Autodesk Inventor part; units mm, degrees
(part 2 of 2)
  spline S266 degree 2 poles (0.3678, -0.7093) (0.2402, -0.5675) (0.1065, -0.294) (0.1065, -0.14) knots 0 0 0 1 2 2 2
  spline S267 degree 2 poles (0.1065, -0.14) (0.1065, 0.1355) (0.4712, 0.4475) (0.8176, 0.4475) knots 0 0 0 1 2 2 2
  line L239 (0.8176, 0.4475) -> (2.0352, 0.4475)
  line L240 (2.831, -11.0699) -> (2.831, -12.2328)
  line L241 (2.831, -12.2328) -> (3.536, -12.2328)
  line L242 (3.536, -12.2328) -> (3.536, -11.1185)
  line L243 (3.536, -11.1185) -> (3.8318, -11.1185)
  line L244 (3.8318, -11.1185) -> (3.8318, -12.2328)
  line L245 (3.8318, -12.2328) -> (5.0352, -12.2328)
  line L246 (5.0352, -12.2328) -> (5.0352, -12.565)
  line L247 (5.0352, -12.565) -> (2.5352, -12.565)
  line L248 (2.5352, -12.565) -> (2.5352, -11.0699)
  line L249 (2.5352, -11.0699) -> (2.831, -11.0699)
  line L250 (5.0352, -10.4743) -> (5.0352, -10.7903)
  line L251 (5.0352, -10.7903) -> (3.1592, -10.7903)
  line L252 (3.1592, -10.7903) -> (3.1592, -10.4743)
  line L253 (3.1592, -10.4743) -> (5.0352, -10.4743)
  line L254 (2.8472, -10.452) -> (2.8472, -10.8106)
  line L255 (2.8472, -10.8106) -> (2.519, -10.8106)
  line L256 (2.519, -10.8106) -> (2.519, -10.452)
  line L257 (2.519, -10.452) -> (2.8472, -10.452)
  line L258 (5.0352, -9.6882) -> (5.0352, -10.0043)
  line L259 (5.0352, -10.0043) -> (2.4238, -10.0043)
  line L260 (2.4238, -10.0043) -> (2.4238, -9.6882)
  line L261 (2.4238, -9.6882) -> (5.0352, -9.6882)
  line L262 (5.0352, -8.9022) -> (5.0352, -9.2182)
  line L263 (5.0352, -9.2182) -> (3.1592, -9.2182)
  line L264 (3.1592, -9.2182) -> (3.1592, -8.9022)
  line L265 (3.1592, -8.9022) -> (5.0352, -8.9022)
  line L266 (2.8472, -8.8799) -> (2.8472, -9.2385)
  line L267 (2.8472, -9.2385) -> (2.519, -9.2385)
  line L268 (2.519, -9.2385) -> (2.519, -8.8799)
  line L269 (2.519, -8.8799) -> (2.8472, -8.8799)
  spline S268 degree 2 poles (4.0465, -6.8661) (4.5165, -6.8661) (5.0716, -7.3138) (5.0716, -7.6562) knots 0 0 0 1 2 2 2
  spline S269 degree 2 poles (5.0716, -7.6562) (5.0716, -7.796) (5.0068, -8.0108) (4.94, -8.1222) knots 0 0 0 1 2 2 2
  line L270 (4.94, -8.1222) -> (5.726, -8.1222)
  line L271 (5.726, -8.1222) -> (5.726, -8.4382)
  line L272 (5.726, -8.4382) -> (3.1592, -8.4382)
  line L273 (3.1592, -8.4382) -> (3.1592, -8.1222)
  line L274 (3.1592, -8.1222) -> (3.3557, -8.1222)
  spline S270 degree 2 poles (3.3557, -8.1222) (3.2483, -8.0047) (3.1065, -7.717) (3.1065, -7.5488) knots 0 0 0 1 2 2 2
  spline S271 degree 2 poles (3.1065, -7.5488) (3.1065, -7.2267) (3.617, -6.8661) (4.0465, -6.8661) knots 0 0 0 1 2 2 2
  spline S272 degree 2 poles (4.083, -7.1923) (3.7609, -7.1923) (3.4063, -7.3969) (3.4063, -7.6258) knots 0 0 0 1 2 2 2
  spline S273 degree 2 poles (3.4063, -7.6258) (3.4063, -7.7595) (3.5259, -8.0108) (3.6191, -8.1222) knots 0 0 0 1 2 2 2
  line L275 (3.6191, -8.1222) -> (4.6847, -8.1222)
  spline S274 degree 2 poles (4.6847, -8.1222) (4.7434, -7.9986) (4.788, -7.8223) (4.788, -7.7089) knots 0 0 0 1 2 2 2
  spline S275 degree 2 poles (4.788, -7.7089) (4.788, -7.4638) (4.4274, -7.1923) (4.083, -7.1923) knots 0 0 0 1 2 2 2
  line L276 (5.0352, -4.984) -> (5.0352, -5.3993)
  line L277 (5.0352, -5.3993) -> (4.1296, -6.0962)
  line L278 (4.1296, -6.0962) -> (4.2511, -6.2219)
  line L279 (4.2511, -6.2219) -> (5.0352, -6.2219)
  line L280 (5.0352, -6.2219) -> (5.0352, -6.5379)
  line L281 (5.0352, -6.5379) -> (2.4238, -6.5379)
  line L282 (2.4238, -6.5379) -> (2.4238, -6.2219)
  line L283 (2.4238, -6.2219) -> (3.9513, -6.2219)
  line L284 (3.9513, -6.2219) -> (3.1592, -5.4804)
  line L285 (3.1592, -5.4804) -> (3.1592, -5.0873)
  line L286 (3.1592, -5.0873) -> (3.9432, -5.8572)
  line L287 (3.9432, -5.8572) -> (5.0352, -4.984)
  spline S276 degree 2 poles (4.0972, -3.2843) (4.5712, -3.2843) (5.0879, -3.7401) (5.0879, -4.121) knots 0 0 0 1 2 2 2
  spline S277 degree 2 poles (5.0879, -4.121) (5.0879, -4.512) (4.555, -4.9597) (4.0972, -4.9597) knots 0 0 0 1 2 2 2
  spline S278 degree 2 poles (4.0972, -4.9597) (3.6272, -4.9597) (3.1065, -4.4978) (3.1065, -4.121) knots 0 0 0 1 2 2 2
  spline S279 degree 2 poles (3.1065, -4.121) (3.1065, -3.7401) (3.6251, -3.2843) (4.0972, -3.2843) knots 0 0 0 1 2 2 2
  spline S280 degree 2 poles (4.0972, -3.6104) (3.7325, -3.6104) (3.378, -3.8758) (3.378, -4.121) knots 0 0 0 1 2 2 2
  spline S281 degree 2 poles (3.378, -4.121) (3.378, -4.3661) (3.7325, -4.6335) (4.0972, -4.6335) knots 0 0 0 1 2 2 2
  spline S282 degree 2 poles (4.0972, -4.6335) (4.4517, -4.6335) (4.8164, -4.3661) (4.8164, -4.121) knots 0 0 0 1 2 2 2
  spline S283 degree 2 poles (4.8164, -4.121) (4.8164, -3.8779) (4.4578, -3.6104) (4.0972, -3.6104) knots 0 0 0 1 2 2 2
  line L288 (3.1592, -0.687) -> (5.0352, -1.1631)
  line L289 (5.0352, -1.1631) -> (5.0352, -1.4548)
  line L290 (5.0352, -1.4548) -> (3.5887, -1.9127)
  line L291 (3.5887, -1.9127) -> (5.0352, -2.3685)
  line L292 (5.0352, -2.3685) -> (5.0352, -2.6582)
  line L293 (5.0352, -2.6582) -> (3.1592, -3.1384)
  line L294 (3.1592, -3.1384) -> (3.1592, -2.8102)
  line L295 (3.1592, -2.8102) -> (4.6118, -2.4779)
  line L296 (4.6118, -2.4779) -> (3.1592, -2.0343)
  line L297 (3.1592, -2.0343) -> (3.1592, -1.7729)
  line L298 (3.1592, -1.7729) -> (4.6118, -1.3171)
  line L299 (4.6118, -1.3171) -> (3.1592, -1.0051)
  line L300 (3.1592, -1.0051) -> (3.1592, -0.687)
  spline S284 degree 2 poles (5.0797, 0.097) (5.0797, -0.0914) (4.9785, -0.4176) (4.9217, -0.5249) knots 0 0 0 1 2 2 2
  line L301 (4.9217, -0.5249) -> (4.5672, -0.5249)
  line L302 (4.5672, -0.5249) -> (4.5672, -0.5087)
  spline S285 degree 2 poles (4.5672, -0.5087) (4.5996, -0.4682) (4.6766, -0.3588) (4.7191, -0.2676) knots 0 0 0 1 2 2 2
  spline S286 degree 2 poles (4.7191, -0.2676) (4.7576, -0.1886) (4.8144, 0.0059) (4.8144, 0.1092) knots 0 0 0 1 2 2 2
  spline S287 degree 2 poles (4.8144, 0.1092) (4.8144, 0.1841) (4.7799, 0.3563) (4.7515, 0.3969) knots 0 0 0 1 2 2 2
  spline S288 degree 2 poles (4.7515, 0.3969) (4.7131, 0.4556) (4.6259, 0.5083) (4.5368, 0.5083) knots 0 0 0 1 2 2 2
  spline S289 degree 2 poles (4.5368, 0.5083) (4.4254, 0.5083) (4.3099, 0.3867) (4.2714, 0.2307) knots 0 0 0 1 2 2 2
  spline S290 degree 2 poles (4.2714, 0.2307) (4.2572, 0.17) (4.2167, -0.0245) (4.1944, -0.1076) knots 0 0 0 1 2 2 2
  spline S291 degree 2 poles (4.1944, -0.1076) (4.1316, -0.3223) (3.8723, -0.5168) (3.6879, -0.5168) knots 0 0 0 1 2 2 2
  spline S292 degree 2 poles (3.6879, -0.5168) (3.4327, -0.5168) (3.1146, -0.1339) (3.1146, 0.1821) knots 0 0 0 1 2 2 2
  spline S293 degree 2 poles (3.1146, 0.1821) (3.1146, 0.3381) (3.1916, 0.6542) (3.2503, 0.7615) knots 0 0 0 1 2 2 2
  line L303 (3.2503, 0.7615) -> (3.5887, 0.7615)
  line L304 (3.5887, 0.7615) -> (3.5887, 0.7453)
  spline S294 degree 2 poles (3.5887, 0.7453) (3.4914, 0.6238) (3.38, 0.328) (3.38, 0.176) knots 0 0 0 1 2 2 2
  spline S295 degree 2 poles (3.38, 0.176) (3.38, 0.02) (3.5117, -0.1947) (3.6434, -0.1947) knots 0 0 0 1 2 2 2
  spline S296 degree 2 poles (3.6434, -0.1947) (3.7629, -0.1947) (3.8784, -0.0671) (3.9148, 0.0747) knots 0 0 0 1 2 2 2
  spline S297 degree 2 poles (3.9148, 0.0747) (3.9331, 0.1436) (3.9695, 0.3179) (3.9918, 0.4131) knots 0 0 0 1 2 2 2
  spline S298 degree 2 poles (3.9918, 0.4131) (4.0445, 0.6197) (4.2856, 0.8304) (4.4943, 0.8304) knots 0 0 0 1 2 2 2
  spline S299 degree 2 poles (4.4943, 0.8304) (4.6158, 0.8304) (4.8306, 0.7352) (4.9096, 0.642) knots 0 0 0 1 2 2 2
  spline S300 degree 2 poles (4.9096, 0.642) (4.9926, 0.5427) (5.0797, 0.2895) (5.0797, 0.097) knots 0 0 0 1 2 2 2
  line L305 (5.0352, 2.6781) -> (5.0352, 2.2627)
  line L306 (5.0352, 2.2627) -> (4.1296, 1.5658)
  line L307 (4.1296, 1.5658) -> (4.2511, 1.4402)
  line L308 (4.2511, 1.4402) -> (5.0352, 1.4402)
  line L309 (5.0352, 1.4402) -> (5.0352, 1.1242)
  line L310 (5.0352, 1.1242) -> (2.4238, 1.1242)
  line L311 (2.4238, 1.1242) -> (2.4238, 1.4402)
  line L312 (2.4238, 1.4402) -> (3.9513, 1.4402)
  line L313 (3.9513, 1.4402) -> (3.1592, 2.1817)
  line L314 (3.1592, 2.1817) -> (3.1592, 2.5747)
  line L315 (3.1592, 2.5747) -> (3.9432, 1.8049)
  line L316 (3.9432, 1.8049) -> (5.0352, 2.6781)
  line L317 (5.0352, 3.1582) -> (5.0352, 2.8422)
  line L318 (5.0352, 2.8422) -> (3.1592, 2.8422)
  line L319 (3.1592, 2.8422) -> (3.1592, 3.1582)
  line L320 (3.1592, 3.1582) -> (5.0352, 3.1582)
  line L321 (2.8472, 3.1805) -> (2.8472, 2.8219)
  line L322 (2.8472, 2.8219) -> (2.519, 2.8219)
  line L323 (2.519, 2.8219) -> (2.519, 3.1805)
  line L324 (2.519, 3.1805) -> (2.8472, 3.1805)
  line L325 (10.2664, -10.4256) -> (10.2664, -10.8571)
  line L326 (10.2664, -10.8571) -> (9.2716, -11.6472)
  line L327 (9.2716, -11.6472) -> (9.2716, -12.0281)
  line L328 (9.2716, -12.0281) -> (10.2664, -12.0281)
  line L329 (10.2664, -12.0281) -> (10.2664, -12.3604)
  line L330 (10.2664, -12.3604) -> (7.7664, -12.3604)
  line L331 (7.7664, -12.3604) -> (7.7664, -11.7161)
  spline S301 degree 2 poles (7.7664, -11.7161) (7.7664, -11.5014) (7.8129, -11.2117) (7.898, -11.08) knots 0 0 0 1 2 2 2
  spline S302 degree 2 poles (7.898, -11.08) (7.9831, -10.9483) (8.2485, -10.7963) (8.445, -10.7963) knots 0 0 0 1 2 2 2
  spline S303 degree 2 poles (8.445, -10.7963) (8.7185, -10.7963) (9.0893, -11.0759) (9.1784, -11.315) knots 0 0 0 1 2 2 2
  line L332 (9.1784, -11.315) -> (10.2664, -10.4256)
  spline S304 degree 2 poles (8.4714, -11.1428) (8.362, -11.1428) (8.1938, -11.2198) (8.1391, -11.3008) knots 0 0 0 1 2 2 2
  spline S305 degree 2 poles (8.1391, -11.3008) (8.0925, -11.3717) (8.054, -11.5601) (8.054, -11.6979) knots 0 0 0 1 2 2 2
  line L333 (8.054, -11.6979) -> (8.054, -12.0281)
  line L334 (8.054, -12.0281) -> (8.9941, -12.0281)
  line L335 (8.9941, -12.0281) -> (8.9941, -11.7364)
  spline S306 degree 2 poles (8.9941, -11.7364) (8.9941, -11.5925) (8.9434, -11.3636) (8.8644, -11.2846) knots 0 0 0 1 2 2 2
  spline S307 degree 2 poles (8.8644, -11.2846) (8.7955, -11.2117) (8.601, -11.1428) (8.4714, -11.1428) knots 0 0 0 1 2 2 2
  spline S308 degree 2 poles (8.052, -8.4584) (8.2181, -8.3166) (8.7044, -8.1586) (9.0164, -8.1586) knots 0 0 0 1 2 2 2
  spline S309 degree 2 poles (9.0164, -8.1586) (9.3202, -8.1586) (9.8125, -8.3126) (9.9787, -8.4584) knots 0 0 0 1 2 2 2
  spline S310 degree 2 poles (9.9787, -8.4584) (10.1529, -8.6124) (10.319, -9.0196) (10.319, -9.2647) knots 0 0 0 1 2 2 2
  spline S311 degree 2 poles (10.319, -9.2647) (10.319, -9.518) (10.1468, -9.9232) (9.9787, -10.0711) knots 0 0 0 1 2 2 2
  spline S312 degree 2 poles (9.9787, -10.0711) (9.8125, -10.2149) (9.3243, -10.3689) (9.0164, -10.3689) knots 0 0 0 1 2 2 2
  spline S313 degree 2 poles (9.0164, -10.3689) (8.7023, -10.3689) (8.2242, -10.2129) (8.052, -10.069) knots 0 0 0 1 2 2 2
  spline S314 degree 2 poles (8.052, -10.069) (7.8859, -9.9232) (7.7137, -9.516) (7.7137, -9.2647) knots 0 0 0 1 2 2 2
  spline S315 degree 2 poles (7.7137, -9.2647) (7.7137, -9.0095) (7.892, -8.6002) (8.052, -8.4584) knots 0 0 0 1 2 2 2
  spline S316 degree 2 poles (9.0164, -8.505) (8.7692, -8.505) (8.3863, -8.6124) (8.2607, -8.7096) knots 0 0 0 1 2 2 2
  spline S317 degree 2 poles (8.2607, -8.7096) (8.131, -8.8089) (8.0014, -9.0885) (8.0014, -9.2627) knots 0 0 0 1 2 2 2
  spline S318 degree 2 poles (8.0014, -9.2627) (8.0014, -9.443) (8.127, -9.7145) (8.2607, -9.8178) knots 0 0 0 1 2 2 2
  spline S319 degree 2 poles (8.2607, -9.8178) (8.3883, -9.9171) (8.7732, -10.0224) (9.0164, -10.0224) knots 0 0 0 1 2 2 2
  spline S320 degree 2 poles (9.0164, -10.0224) (9.5087, -10.0224) (10.0313, -9.6092) (10.0313, -9.2627) knots 0 0 0 1 2 2 2
  spline S321 degree 2 poles (10.0313, -9.2627) (10.0313, -8.9163) (9.5087, -8.505) (9.0164, -8.505) knots 0 0 0 1 2 2 2
  spline S322 degree 2 poles (9.4985, -6.0982) (9.6849, -6.0982) (9.9706, -6.24) (10.0638, -6.3575) knots 0 0 0 1 2 2 2
  spline S323 degree 2 poles (10.0638, -6.3575) (10.1732, -6.4993) (10.2664, -6.8215) (10.2664, -7.0767) knots 0 0 0 1 2 2 2
  line L336 (10.2664, -7.0767) -> (10.2664, -7.7939)
  line L337 (10.2664, -7.7939) -> (7.7664, -7.7939)
  line L338 (7.7664, -7.7939) -> (7.7664, -7.1314)
  spline S324 degree 2 poles (7.7664, -7.1314) (7.7664, -6.864) (7.8008, -6.5966) (7.8676, -6.475) knots 0 0 0 1 2 2 2
  spline S325 degree 2 poles (7.8676, -6.475) (7.9386, -6.3393) (8.1715, -6.2157) (8.3296, -6.2157) knots 0 0 0 1 2 2 2
  spline S326 degree 2 poles (8.3296, -6.2157) (8.5058, -6.2157) (8.7854, -6.4021) (8.8644, -6.5662) knots 0 0 0 1 2 2 2
  line L339 (8.8644, -6.5662) -> (8.8766, -6.5662)
  spline S327 degree 2 poles (8.8766, -6.5662) (8.9373, -6.3433) (9.2595, -6.0982) (9.4985, -6.0982) knots 0 0 0 1 2 2 2
  spline S328 degree 2 poles (9.5127, -6.4446) (9.3709, -6.4446) (9.1886, -6.5257) (9.1237, -6.6472) knots 0 0 0 1 2 2 2
  spline S329 degree 2 poles (9.1237, -6.6472) (9.0832, -6.7263) (9.0589, -6.9126) (9.0589, -7.0848) knots 0 0 0 1 2 2 2
  line L340 (9.0589, -7.0848) -> (9.0589, -7.4617)
  line L341 (9.0589, -7.4617) -> (9.9827, -7.4617)
  line L342 (9.9827, -7.4617) -> (9.9827, -7.1922)
  spline S330 degree 2 poles (9.9827, -7.1922) (9.9827, -6.9734) (9.9422, -6.7222) (9.8774, -6.625) knots 0 0 0 1 2 2 2
  spline S331 degree 2 poles (9.8774, -6.625) (9.8105, -6.5318) (9.6444, -6.4446) (9.5127, -6.4446) knots 0 0 0 1 2 2 2
  spline S332 degree 2 poles (8.3762, -6.5622) (8.287, -6.5622) (8.1533, -6.6229) (8.1148, -6.6898) knots 0 0 0 1 2 2 2
  spline S333 degree 2 poles (8.1148, -6.6898) (8.0702, -6.7708) (8.05, -6.9673) (8.05, -7.1436) knots 0 0 0 1 2 2 2
  line L343 (8.05, -7.1436) -> (8.05, -7.4617)
  line L344 (8.05, -7.4617) -> (8.7813, -7.4617)
  line L345 (8.7813, -7.4617) -> (8.7813, -7.0848)
  spline S334 degree 2 poles (8.7813, -7.0848) (8.7813, -6.9288) (8.7489, -6.781) (8.6983, -6.7019) knots 0 0 0 1 2 2 2
  spline S335 degree 2 poles (8.6983, -6.7019) (8.6497, -6.625) (8.4937, -6.5622) (8.3762, -6.5622) knots 0 0 0 1 2 2 2
  spline S336 degree 2 poles (8.052, -3.9993) (8.2181, -3.8575) (8.7044, -3.6995) (9.0164, -3.6995) knots 0 0 0 1 2 2 2
  spline S337 degree 2 poles (9.0164, -3.6995) (9.3202, -3.6995) (9.8125, -3.8535) (9.9787, -3.9993) knots 0 0 0 1 2 2 2
  spline S338 degree 2 poles (9.9787, -3.9993) (10.1529, -4.1533) (10.319, -4.5605) (10.319, -4.8057) knots 0 0 0 1 2 2 2
  spline S339 degree 2 poles (10.319, -4.8057) (10.319, -5.0589) (10.1468, -5.4641) (9.9787, -5.612) knots 0 0 0 1 2 2 2
  spline S340 degree 2 poles (9.9787, -5.612) (9.8125, -5.7558) (9.3243, -5.9098) (9.0164, -5.9098) knots 0 0 0 1 2 2 2
  spline S341 degree 2 poles (9.0164, -5.9098) (8.7023, -5.9098) (8.2242, -5.7538) (8.052, -5.61) knots 0 0 0 1 2 2 2
  spline S342 degree 2 poles (8.052, -5.61) (7.8859, -5.4641) (7.7137, -5.0569) (7.7137, -4.8057) knots 0 0 0 1 2 2 2
  spline S343 degree 2 poles (7.7137, -4.8057) (7.7137, -4.5504) (7.892, -4.1412) (8.052, -3.9993) knots 0 0 0 1 2 2 2
  spline S344 degree 2 poles (9.0164, -4.0459) (8.7692, -4.0459) (8.3863, -4.1533) (8.2607, -4.2506) knots 0 0 0 1 2 2 2
  spline S345 degree 2 poles (8.2607, -4.2506) (8.131, -4.3498) (8.0014, -4.6294) (8.0014, -4.8036) knots 0 0 0 1 2 2 2
  spline S346 degree 2 poles (8.0014, -4.8036) (8.0014, -4.9839) (8.127, -5.2554) (8.2607, -5.3587) knots 0 0 0 1 2 2 2
  spline S347 degree 2 poles (8.2607, -5.3587) (8.3883, -5.458) (8.7732, -5.5634) (9.0164, -5.5634) knots 0 0 0 1 2 2 2
  spline S348 degree 2 poles (9.0164, -5.5634) (9.5087, -5.5634) (10.0313, -5.1501) (10.0313, -4.8036) knots 0 0 0 1 2 2 2
  spline S349 degree 2 poles (10.0313, -4.8036) (10.0313, -4.4572) (9.5087, -4.0459) (9.0164, -4.0459) knots 0 0 0 1 2 2 2
  line L346 (10.2664, -2.4637) -> (10.2664, -3.4321)
  line L347 (10.2664, -3.4321) -> (10.0111, -3.4321)
  line L348 (10.0111, -3.4321) -> (10.0111, -3.114)
  line L349 (10.0111, -3.114) -> (8.0216, -3.114)
  line L350 (8.0216, -3.114) -> (8.0216, -3.4321)
  line L351 (8.0216, -3.4321) -> (7.7664, -3.4321)
  line L352 (7.7664, -3.4321) -> (7.7664, -2.4637)
  line L353 (7.7664, -2.4637) -> (8.0216, -2.4637)
  line L354 (8.0216, -2.4637) -> (8.0216, -2.7818)
  line L355 (8.0216, -2.7818) -> (10.0111, -2.7818)
  line L356 (10.0111, -2.7818) -> (10.0111, -2.4637)
  line L357 (10.0111, -2.4637) -> (10.2664, -2.4637)
  line L358 (10.2664, -0.6039) -> (10.2664, -2.0524)
  line L359 (10.2664, -2.0524) -> (7.7664, -2.0524)
  line L360 (7.7664, -2.0524) -> (7.7664, -1.7202)
  line L361 (7.7664, -1.7202) -> (9.9706, -1.7202)
  line L362 (9.9706, -1.7202) -> (9.9706, -0.6039)
  line L363 (9.9706, -0.6039) -> (10.2664, -0.6039)
  spline S350 degree 2 poles (8.052, 1.4261) (8.2181, 1.5679) (8.7044, 1.7259) (9.0164, 1.7259) knots 0 0 0 1 2 2 2
  spline S351 degree 2 poles (9.0164, 1.7259) (9.3202, 1.7259) (9.8125, 1.572) (9.9787, 1.4261) knots 0 0 0 1 2 2 2
  spline S352 degree 2 poles (9.9787, 1.4261) (10.1529, 1.2721) (10.319, 0.8649) (10.319, 0.6198) knots 0 0 0 1 2 2 2
  spline S353 degree 2 poles (10.319, 0.6198) (10.319, 0.3665) (10.1468, -0.0386) (9.9787, -0.1865) knots 0 0 0 1 2 2 2
  spline S354 degree 2 poles (9.9787, -0.1865) (9.8125, -0.3304) (9.3243, -0.4844) (9.0164, -0.4844) knots 0 0 0 1 2 2 2
  spline S355 degree 2 poles (9.0164, -0.4844) (8.7023, -0.4844) (8.2242, -0.3284) (8.052, -0.1845) knots 0 0 0 1 2 2 2
  spline S356 degree 2 poles (8.052, -0.1845) (7.8859, -0.0386) (7.7137, 0.3686) (7.7137, 0.6198) knots 0 0 0 1 2 2 2
  spline S357 degree 2 poles (7.7137, 0.6198) (7.7137, 0.875) (7.892, 1.2843) (8.052, 1.4261) knots 0 0 0 1 2 2 2
  spline S358 degree 2 poles (9.0164, 1.3795) (8.7692, 1.3795) (8.3863, 1.2721) (8.2607, 1.1749) knots 0 0 0 1 2 2 2
  spline S359 degree 2 poles (8.2607, 1.1749) (8.131, 1.0756) (8.0014, 0.796) (8.0014, 0.6218) knots 0 0 0 1 2 2 2
  spline S360 degree 2 poles (8.0014, 0.6218) (8.0014, 0.4415) (8.127, 0.17) (8.2607, 0.0667) knots 0 0 0 1 2 2 2
  spline S361 degree 2 poles (8.2607, 0.0667) (8.3883, -0.0326) (8.7732, -0.1379) (9.0164, -0.1379) knots 0 0 0 1 2 2 2
  spline S362 degree 2 poles (9.0164, -0.1379) (9.5087, -0.1379) (10.0313, 0.2754) (10.0313, 0.6218) knots 0 0 0 1 2 2 2
  spline S363 degree 2 poles (10.0313, 0.6218) (10.0313, 0.9682) (9.5087, 1.3795) (9.0164, 1.3795) knots 0 0 0 1 2 2 2
  spline S364 degree 2 poles (6.6213, 11.6859) (6.6213, 11.4205) (6.4593, 10.9809) (6.2952, 10.8229) knots 0 0 0 1 2 2 2
  spline S365 degree 2 poles (6.2952, 10.8229) (6.129, 10.6648) (5.6388, 10.4967) (5.3207, 10.4967) knots 0 0 0 1 2 2 2
  spline S366 degree 2 poles (5.3207, 10.4967) (5.0188, 10.4967) (4.5407, 10.6669) (4.3705, 10.8249) knots 0 0 0 1 2 2 2
  spline S367 degree 2 poles (4.3705, 10.8249) (4.2064, 10.9768) (4.0281, 11.4225) (4.0281, 11.6879) knots 0 0 0 1 2 2 2
  spline S368 degree 2 poles (4.0281, 11.6879) (4.0281, 11.8156) (4.0646, 12.0465) (4.097, 12.1519) knots 0 0 0 1 2 2 2
  spline S369 degree 2 poles (4.097, 12.1519) (4.1213, 12.237) (4.2105, 12.4436) (4.2429, 12.5064) knots 0 0 0 1 2 2 2
  line L364 (4.2429, 12.5064) -> (4.644, 12.5064)
  line L365 (4.644, 12.5064) -> (4.644, 12.478)
  spline S370 degree 2 poles (4.644, 12.478) (4.5893, 12.4152) (4.49, 12.2836) (4.4333, 12.162) knots 0 0 0 1 2 2 2
  spline S371 degree 2 poles (4.4333, 12.162) (4.3827, 12.0607) (4.3158, 11.7994) (4.3158, 11.6494) knots 0 0 0 1 2 2 2
  spline S372 degree 2 poles (4.3158, 11.6494) (4.3158, 11.2888) (4.8588, 10.8431) (5.3105, 10.8431) knots 0 0 0 1 2 2 2
  spline S373 degree 2 poles (5.3105, 10.8431) (5.5618, 10.8431) (5.9386, 10.9606) (6.0682, 11.072) knots 0 0 0 1 2 2 2
  spline S374 degree 2 poles (6.0682, 11.072) (6.1979, 11.1794) (6.3336, 11.4833) (6.3336, 11.6738) knots 0 0 0 1 2 2 2
  spline S375 degree 2 poles (6.3336, 11.6738) (6.3336, 11.8135) (6.2931, 12.0931) (6.2526, 12.1883) knots 0 0 0 1 2 2 2
  line L366 (6.2526, 12.1883) -> (5.6063, 12.1883)
  line L367 (5.6063, 12.1883) -> (5.6063, 11.6089)
  line L368 (5.6063, 11.6089) -> (5.3146, 11.6089)
  line L369 (5.3146, 11.6089) -> (5.3146, 12.5165)
  line L370 (5.3146, 12.5165) -> (6.4066, 12.5165)
  spline S376 degree 2 poles (6.4066, 12.5165) (6.4349, 12.4537) (6.5221, 12.239) (6.5484, 12.1478) knots 0 0 0 1 2 2 2
  spline S377 degree 2 poles (6.5484, 12.1478) (6.5849, 12.0242) (6.6213, 11.8257) (6.6213, 11.6859) knots 0 0 0 1 2 2 2
  line L371 (6.5727, 14.7228) -> (6.5727, 14.35)
  line L372 (6.5727, 14.35) -> (4.4171, 13.2438)
  line L373 (4.4171, 13.2438) -> (6.5727, 13.2438)
  line L374 (6.5727, 13.2438) -> (6.5727, 12.9339)
  line L375 (6.5727, 12.9339) -> (4.0727, 12.9339)
  line L376 (4.0727, 12.9339) -> (4.0727, 13.4059)
  line L377 (4.0727, 13.4059) -> (6.052, 14.4128)
  line L378 (6.052, 14.4128) -> (4.0727, 14.4128)
  line L379 (4.0727, 14.4128) -> (4.0727, 14.7228)
  line L380 (4.0727, 14.7228) -> (6.5727, 14.7228)
  spline S378 degree 2 poles (5.3247, 17.2005) (5.6671, 17.2005) (6.2182, 16.9229) (6.3721, 16.69) knots 0 0 0 1 2 2 2
  spline S379 degree 2 poles (6.3721, 16.69) (6.4917, 16.4995) (6.5727, 16.1085) (6.5727, 15.8046) knots 0 0 0 1 2 2 2
  line L381 (6.5727, 15.8046) -> (6.5727, 15.2293)
  line L382 (6.5727, 15.2293) -> (4.0727, 15.2293)
  line L383 (4.0727, 15.2293) -> (4.0727, 15.7985)
  spline S380 degree 2 poles (4.0727, 15.7985) (4.0727, 16.1511) (4.1781, 16.5522) (4.2712, 16.694) knots 0 0 0 1 2 2 2
  spline S381 degree 2 poles (4.2712, 16.694) (4.4313, 16.9351) (4.9601, 17.2005) (5.3247, 17.2005) knots 0 0 0 1 2 2 2
  spline S382 degree 2 poles (5.3207, 16.8541) (5.033, 16.8541) (4.6258, 16.6636) (4.5103, 16.4752) knots 0 0 0 1 2 2 2
  spline S383 degree 2 poles (4.5103, 16.4752) (4.4313, 16.3415) (4.3604, 16.0396) (4.3604, 15.8148) knots 0 0 0 1 2 2 2
  line L384 (4.3604, 15.8148) -> (4.3604, 15.5615)
  line L385 (4.3604, 15.5615) -> (6.285, 15.5615)
  line L386 (6.285, 15.5615) -> (6.285, 15.8148)
  spline S384 degree 2 poles (6.285, 15.8148) (6.285, 16.0356) (6.2141, 16.3699) (6.1189, 16.5056) knots 0 0 0 1 2 2 2
  spline S385 degree 2 poles (6.1189, 16.5056) (6.0014, 16.6798) (5.6124, 16.8541) (5.3207, 16.8541) knots 0 0 0 1 2 2 2
  line L387 (9.2727, 12.6817) -> (7.0685, 12.6817)
  line L388 (7.0685, 12.6817) -> (7.0685, 11.8429)
  line L389 (7.0685, 11.8429) -> (6.7727, 11.8429)
  line L390 (6.7727, 11.8429) -> (6.7727, 13.8526)
  line L391 (6.7727, 13.8526) -> (7.0685, 13.8526)
  line L392 (7.0685, 13.8526) -> (7.0685, 13.0139)
  line L393 (7.0685, 13.0139) -> (9.2727, 13.0139)
  line L394 (9.2727, 13.0139) -> (9.2727, 12.6817)
  line L395 (9.2727, 15.834) -> (9.2727, 15.4531)
  line L396 (9.2727, 15.4531) -> (8.2759, 14.8453)
  line L397 (8.2759, 14.8453) -> (9.2727, 14.2254)
  line L398 (9.2727, 14.2254) -> (9.2727, 13.8668)
  line L399 (9.2727, 13.8668) -> (8.0207, 14.663)
  line L400 (8.0207, 14.663) -> (6.7727, 13.8911)
  line L401 (6.7727, 13.8911) -> (6.7727, 14.272)
  line L402 (6.7727, 14.272) -> (7.7512, 14.8676)
  line L403 (7.7512, 14.8676) -> (6.7727, 15.4754)
  line L404 (6.7727, 15.4754) -> (6.7727, 15.834)
  line L405 (6.7727, 15.834) -> (8.0045, 15.052)
  line L406 (8.0045, 15.052) -> (9.2727, 15.834)
  line L407 (11.9727, 13.9701) -> (11.9727, 13.5386)
  line L408 (11.9727, 13.5386) -> (10.978, 12.7485)
  line L409 (10.978, 12.7485) -> (10.978, 12.3676)
  line L410 (10.978, 12.3676) -> (11.9727, 12.3676)
  line L411 (11.9727, 12.3676) -> (11.9727, 12.0354)
  line L412 (11.9727, 12.0354) -> (9.4727, 12.0354)
  line L413 (9.4727, 12.0354) -> (9.4727, 12.6796)
  spline S386 degree 2 poles (9.4727, 12.6796) (9.4727, 12.8944) (9.5193, 13.1841) (9.6044, 13.3158) knots 0 0 0 1 2 2 2
  spline S387 degree 2 poles (9.6044, 13.3158) (9.6895, 13.4475) (9.9549, 13.5994) (10.1514, 13.5994) knots 0 0 0 1 2 2 2
  spline S388 degree 2 poles (10.1514, 13.5994) (10.4249, 13.5994) (10.7956, 13.3198) (10.8848, 13.0808) knots 0 0 0 1 2 2 2
  line L414 (10.8848, 13.0808) -> (11.9727, 13.9701)
  spline S389 degree 2 poles (10.1777, 13.253) (10.0683, 13.253) (9.9002, 13.176) (9.8455, 13.0949) knots 0 0 0 1 2 2 2
  spline S390 degree 2 poles (9.8455, 13.0949) (9.7989, 13.024) (9.7604, 12.8356) (9.7604, 12.6979) knots 0 0 0 1 2 2 2
  line L415 (9.7604, 12.6979) -> (9.7604, 12.3676)
  line L416 (9.7604, 12.3676) -> (10.7004, 12.3676)
  line L417 (10.7004, 12.3676) -> (10.7004, 12.6594)
  spline S391 degree 2 poles (10.7004, 12.6594) (10.7004, 12.8032) (10.6498, 13.0321) (10.5708, 13.1111) knots 0 0 0 1 2 2 2
  spline S392 degree 2 poles (10.5708, 13.1111) (10.5019, 13.1841) (10.3074, 13.253) (10.1777, 13.253) knots 0 0 0 1 2 2 2
  line L418 (11.9727, 15.8968) -> (11.9727, 15.5159)
  line L419 (11.9727, 15.5159) -> (10.9759, 14.9082)
  line L420 (10.9759, 14.9082) -> (11.9727, 14.2882)
  line L421 (11.9727, 14.2882) -> (11.9727, 13.9296)
  line L422 (11.9727, 13.9296) -> (10.7207, 14.7258)
  line L423 (10.7207, 14.7258) -> (9.4727, 13.9539)
  line L424 (9.4727, 13.9539) -> (9.4727, 14.3348)
  line L425 (9.4727, 14.3348) -> (10.4512, 14.9304)
  line L426 (10.4512, 14.9304) -> (9.4727, 15.5382)
  line L427 (9.4727, 15.5382) -> (9.4727, 15.8968)
  line L428 (9.4727, 15.8968) -> (10.7045, 15.1148)
  line L429 (10.7045, 15.1148) -> (11.9727, 15.8968)
  spline S393 degree 2 poles (-6.9006, 11.414) (-6.9006, 11.3229) (-6.856, 11.1426) (-6.8215, 11.0554) knots 0 0 0 1 2 2 2
  spline S394 degree 2 poles (-6.8215, 11.0554) (-6.7871, 10.9744) (-6.7142, 10.8549) (-6.6818, 10.8083) knots 0 0 0 1 2 2 2
  line L430 (-6.6818, 10.8083) -> (-6.6818, 10.788)
  line L431 (-6.6818, 10.788) -> (-7.0363, 10.788)
  spline S395 degree 2 poles (-7.0363, 10.788) (-7.095, 10.8974) (-7.1903, 11.2722) (-7.1903, 11.4404) knots 0 0 0 1 2 2 2
  spline S396 degree 2 poles (-7.1903, 11.4404) (-7.1903, 11.6106) (-7.1214, 11.8638) (-7.0484, 11.9671) knots 0 0 0 1 2 2 2
  spline S397 degree 2 poles (-7.0484, 11.9671) (-6.9694, 12.0765) (-6.7405, 12.19) (-6.5865, 12.19) knots 0 0 0 1 2 2 2
  spline S398 degree 2 poles (-6.5865, 12.19) (-6.3799, 12.19) (-6.0679, 11.9185) (-6.0274, 11.7281) knots 0 0 0 1 2 2 2
  line L432 (-6.0274, 11.7281) -> (-6.0031, 11.7281)
  spline S399 degree 2 poles (-6.0031, 11.7281) (-5.9869, 11.8071) (-5.9139, 11.9874) (-5.841, 12.0644) knots 0 0 0 1 2 2 2
  spline S400 degree 2 poles (-5.841, 12.0644) (-5.7701, 12.1413) (-5.5432, 12.2386) (-5.3791, 12.2386) knots 0 0 0 1 2 2 2
  spline S401 degree 2 poles (-5.3791, 12.2386) (-5.2109, 12.2386) (-4.9253, 12.1231) (-4.8159, 12.0178) knots 0 0 0 1 2 2 2
  spline S402 degree 2 poles (-4.8159, 12.0178) (-4.7024, 11.9084) (-4.5849, 11.5984) (-4.5849, 11.4019) knots 0 0 0 1 2 2 2
  spline S403 degree 2 poles (-4.5849, 11.4019) (-4.5849, 11.2135) (-4.6761, 10.8448) (-4.7389, 10.7191) knots 0 0 0 1 2 2 2
  line L433 (-4.7389, 10.7191) -> (-5.0934, 10.7191)
  line L434 (-5.0934, 10.7191) -> (-5.0934, 10.7435)
  spline S404 degree 2 poles (-5.0934, 10.7435) (-5.0164, 10.8488) (-4.8746, 11.2054) (-4.8746, 11.3816) knots 0 0 0 1 2 2 2
  spline S405 degree 2 poles (-4.8746, 11.3816) (-4.8746, 11.4849) (-4.9395, 11.6916) (-5.0144, 11.7605) knots 0 0 0 1 2 2 2
  spline S406 degree 2 poles (-5.0144, 11.7605) (-5.0894, 11.8273) (-5.2677, 11.8982) (-5.4034, 11.8982) knots 0 0 0 1 2 2 2
  spline S407 degree 2 poles (-5.4034, 11.8982) (-5.5391, 11.8982) (-5.7154, 11.8192) (-5.766, 11.7483) knots 0 0 0 1 2 2 2
  spline S408 degree 2 poles (-5.766, 11.7483) (-5.8167, 11.6774) (-5.8552, 11.4849) (-5.8552, 11.3715) knots 0 0 0 1 2 2 2
  line L435 (-5.8552, 11.3715) -> (-5.8552, 11.2297)
  line L436 (-5.8552, 11.2297) -> (-6.1327, 11.2297)
  line L437 (-6.1327, 11.2297) -> (-6.1327, 11.3411)
  spline S409 degree 2 poles (-6.1327, 11.3411) (-6.1327, 11.566) (-6.3475, 11.8496) (-6.5521, 11.8496) knots 0 0 0 1 2 2 2
  spline S410 degree 2 poles (-6.5521, 11.8496) (-6.6473, 11.8496) (-6.7831, 11.7767) (-6.8236, 11.7179) knots 0 0 0 1 2 2 2
  spline S411 degree 2 poles (-6.8236, 11.7179) (-6.8661, 11.6551) (-6.9006, 11.5012) (-6.9006, 11.414) knots 0 0 0 1 2 2 2
  line L438 (-4.6376, 13.1523) -> (-4.6376, 12.7512)
  line L439 (-4.6376, 12.7512) -> (-5.1157, 12.7512)
  line L440 (-5.1157, 12.7512) -> (-5.1157, 13.1523)
  line L441 (-5.1157, 13.1523) -> (-4.6376, 13.1523)
  spline S412 degree 2 poles (-6.9006, 14.3314) (-6.9006, 14.2402) (-6.856, 14.0599) (-6.8215, 13.9728) knots 0 0 0 1 2 2 2
  spline S413 degree 2 poles (-6.8215, 13.9728) (-6.7871, 13.8918) (-6.7142, 13.7722) (-6.6818, 13.7256) knots 0 0 0 1 2 2 2
  line L442 (-6.6818, 13.7256) -> (-6.6818, 13.7054)
  line L443 (-6.6818, 13.7054) -> (-7.0363, 13.7054)
  spline S414 degree 2 poles (-7.0363, 13.7054) (-7.095, 13.8148) (-7.1903, 14.1896) (-7.1903, 14.3577) knots 0 0 0 1 2 2 2
  spline S415 degree 2 poles (-7.1903, 14.3577) (-7.1903, 14.5279) (-7.1214, 14.7811) (-7.0484, 14.8845) knots 0 0 0 1 2 2 2
  spline S416 degree 2 poles (-7.0484, 14.8845) (-6.9694, 14.9939) (-6.7405, 15.1073) (-6.5865, 15.1073) knots 0 0 0 1 2 2 2
  spline S417 degree 2 poles (-6.5865, 15.1073) (-6.3799, 15.1073) (-6.0679, 14.8358) (-6.0274, 14.6454) knots 0 0 0 1 2 2 2
  line L444 (-6.0274, 14.6454) -> (-6.0031, 14.6454)
  spline S418 degree 2 poles (-6.0031, 14.6454) (-5.9869, 14.7244) (-5.9139, 14.9047) (-5.841, 14.9817) knots 0 0 0 1 2 2 2
  spline S419 degree 2 poles (-5.841, 14.9817) (-5.7701, 15.0587) (-5.5432, 15.1559) (-5.3791, 15.1559) knots 0 0 0 1 2 2 2
  spline S420 degree 2 poles (-5.3791, 15.1559) (-5.2109, 15.1559) (-4.9253, 15.0405) (-4.8159, 14.9351) knots 0 0 0 1 2 2 2
  spline S421 degree 2 poles (-4.8159, 14.9351) (-4.7024, 14.8257) (-4.5849, 14.5157) (-4.5849, 14.3192) knots 0 0 0 1 2 2 2
  spline S422 degree 2 poles (-4.5849, 14.3192) (-4.5849, 14.1308) (-4.6761, 13.7621) (-4.7389, 13.6365) knots 0 0 0 1 2 2 2
  line L445 (-4.7389, 13.6365) -> (-5.0934, 13.6365)
  line L446 (-5.0934, 13.6365) -> (-5.0934, 13.6608)
  spline S423 degree 2 poles (-5.0934, 13.6608) (-5.0164, 13.7661) (-4.8746, 14.1227) (-4.8746, 14.299) knots 0 0 0 1 2 2 2
  spline S424 degree 2 poles (-4.8746, 14.299) (-4.8746, 14.4023) (-4.9395, 14.6089) (-5.0144, 14.6778) knots 0 0 0 1 2 2 2
  spline S425 degree 2 poles (-5.0144, 14.6778) (-5.0894, 14.7447) (-5.2677, 14.8156) (-5.4034, 14.8156) knots 0 0 0 1 2 2 2
  spline S426 degree 2 poles (-5.4034, 14.8156) (-5.5391, 14.8156) (-5.7154, 14.7366) (-5.766, 14.6657) knots 0 0 0 1 2 2 2
  spline S427 degree 2 poles (-5.766, 14.6657) (-5.8167, 14.5948) (-5.8552, 14.4023) (-5.8552, 14.2888) knots 0 0 0 1 2 2 2
  line L447 (-5.8552, 14.2888) -> (-5.8552, 14.147)
  line L448 (-5.8552, 14.147) -> (-6.1327, 14.147)
  line L449 (-6.1327, 14.147) -> (-6.1327, 14.2584)
  spline S428 degree 2 poles (-6.1327, 14.2584) (-6.1327, 14.4833) (-6.3475, 14.767) (-6.5521, 14.767) knots 0 0 0 1 2 2 2
  spline S429 degree 2 poles (-6.5521, 14.767) (-6.6473, 14.767) (-6.7831, 14.694) (-6.8236, 14.6353) knots 0 0 0 1 2 2 2
  spline S430 degree 2 poles (-6.8236, 14.6353) (-6.8661, 14.5725) (-6.9006, 14.4185) (-6.9006, 14.3314) knots 0 0 0 1 2 2 2
  line L450 (-6.5136, 17.0522) -> (-4.6376, 16.3452)
  line L451 (-4.6376, 16.3452) -> (-4.6376, 16.0615)
  line L452 (-4.6376, 16.0615) -> (-6.5136, 15.3606)
  line L453 (-6.5136, 15.3606) -> (-6.5136, 15.7029)
  line L454 (-6.5136, 15.7029) -> (-5.0691, 16.2155)
  line L455 (-5.0691, 16.2155) -> (-6.5136, 16.724)
  line L456 (-6.5136, 16.724) -> (-6.5136, 17.0522)
  spline S431 degree 2 poles (-1.889, 11.649) (-1.889, 11.3836) (-2.051, 10.944) (-2.2151, 10.786) knots 0 0 0 1 2 2 2
  spline S432 degree 2 poles (-2.2151, 10.786) (-2.3813, 10.628) (-2.8715, 10.4598) (-3.1896, 10.4598) knots 0 0 0 1 2 2 2
  spline S433 degree 2 poles (-3.1896, 10.4598) (-3.4915, 10.4598) (-3.9696, 10.63) (-4.1398, 10.788) knots 0 0 0 1 2 2 2
  spline S434 degree 2 poles (-4.1398, 10.788) (-4.3039, 10.94) (-4.4822, 11.3857) (-4.4822, 11.6511) knots 0 0 0 1 2 2 2
  spline S435 degree 2 poles (-4.4822, 11.6511) (-4.4822, 11.7787) (-4.4457, 12.0097) (-4.4133, 12.115) knots 0 0 0 1 2 2 2
  spline S436 degree 2 poles (-4.4133, 12.115) (-4.389, 12.2001) (-4.2998, 12.4067) (-4.2674, 12.4695) knots 0 0 0 1 2 2 2
  line L457 (-4.2674, 12.4695) -> (-3.8663, 12.4695)
  line L458 (-3.8663, 12.4695) -> (-3.8663, 12.4412)
  spline S437 degree 2 poles (-3.8663, 12.4412) (-3.921, 12.3784) (-4.0202, 12.2467) (-4.077, 12.1251) knots 0 0 0 1 2 2 2
  spline S438 degree 2 poles (-4.077, 12.1251) (-4.1276, 12.0238) (-4.1945, 11.7625) (-4.1945, 11.6126) knots 0 0 0 1 2 2 2
  spline S439 degree 2 poles (-4.1945, 11.6126) (-4.1945, 11.252) (-3.6515, 10.8063) (-3.1997, 10.8063) knots 0 0 0 1 2 2 2
  spline S440 degree 2 poles (-3.1997, 10.8063) (-2.9485, 10.8063) (-2.5717, 10.9238) (-2.442, 11.0352) knots 0 0 0 1 2 2 2
  spline S441 degree 2 poles (-2.442, 11.0352) (-2.3124, 11.1426) (-2.1766, 11.4465) (-2.1766, 11.6369) knots 0 0 0 1 2 2 2
  spline S442 degree 2 poles (-2.1766, 11.6369) (-2.1766, 11.7767) (-2.2172, 12.0563) (-2.2577, 12.1515) knots 0 0 0 1 2 2 2
  line L459 (-2.2577, 12.1515) -> (-2.904, 12.1515)
  line L460 (-2.904, 12.1515) -> (-2.904, 11.5721)
  line L461 (-2.904, 11.5721) -> (-3.1957, 11.5721)
  line L462 (-3.1957, 11.5721) -> (-3.1957, 12.4797)
  line L463 (-3.1957, 12.4797) -> (-2.1037, 12.4797)
  spline S443 degree 2 poles (-2.1037, 12.4797) (-2.0754, 12.4169) (-1.9882, 12.2021) (-1.9619, 12.111) knots 0 0 0 1 2 2 2
  spline S444 degree 2 poles (-1.9619, 12.111) (-1.9254, 11.9874) (-1.889, 11.7888) (-1.889, 11.649) knots 0 0 0 1 2 2 2
  line L464 (-1.9376, 14.6859) -> (-1.9376, 14.3131)
  line L465 (-1.9376, 14.3131) -> (-4.0932, 13.207)
  line L466 (-4.0932, 13.207) -> (-1.9376, 13.207)
  line L467 (-1.9376, 13.207) -> (-1.9376, 12.897)
  line L468 (-1.9376, 12.897) -> (-4.4376, 12.897)
  line L469 (-4.4376, 12.897) -> (-4.4376, 13.3691)
  line L470 (-4.4376, 13.3691) -> (-2.4583, 14.376)
  line L471 (-2.4583, 14.376) -> (-4.4376, 14.376)
  line L472 (-4.4376, 14.376) -> (-4.4376, 14.6859)
  line L473 (-4.4376, 14.6859) -> (-1.9376, 14.6859)
  spline S445 degree 2 poles (-3.1856, 17.1636) (-2.8432, 17.1636) (-2.2921, 16.8861) (-2.1382, 16.6531) knots 0 0 0 1 2 2 2
  spline S446 degree 2 poles (-2.1382, 16.6531) (-2.0186, 16.4627) (-1.9376, 16.0717) (-1.9376, 15.7678) knots 0 0 0 1 2 2 2
  line L474 (-1.9376, 15.7678) -> (-1.9376, 15.1924)
  line L475 (-1.9376, 15.1924) -> (-4.4376, 15.1924)
  line L476 (-4.4376, 15.1924) -> (-4.4376, 15.7617)
  spline S447 degree 2 poles (-4.4376, 15.7617) (-4.4376, 16.1142) (-4.3322, 16.5153) (-4.239, 16.6571) knots 0 0 0 1 2 2 2
  spline S448 degree 2 poles (-4.239, 16.6571) (-4.079, 16.8982) (-3.5502, 17.1636) (-3.1856, 17.1636) knots 0 0 0 1 2 2 2
  spline S449 degree 2 poles (-3.1896, 16.8172) (-3.4773, 16.8172) (-3.8845, 16.6268) (-4, 16.4383) knots 0 0 0 1 2 2 2
  spline S450 degree 2 poles (-4, 16.4383) (-4.079, 16.3046) (-4.1499, 16.0028) (-4.1499, 15.7779) knots 0 0 0 1 2 2 2
  line L477 (-4.1499, 15.7779) -> (-4.1499, 15.5247)
  line L478 (-4.1499, 15.5247) -> (-2.2253, 15.5247)
  line L479 (-2.2253, 15.5247) -> (-2.2253, 15.7779)
  spline S451 degree 2 poles (-2.2253, 15.7779) (-2.2253, 15.9987) (-2.2962, 16.333) (-2.3914, 16.4687) knots 0 0 0 1 2 2 2
  spline S452 degree 2 poles (-2.3914, 16.4687) (-2.5089, 16.643) (-2.8979, 16.8172) (-3.1896, 16.8172) knots 0 0 0 1 2 2 2
  line L480 (0.7624, 13.1452) -> (0.7624, 12.1768)
  line L481 (0.7624, 12.1768) -> (0.5071, 12.1768)
  line L482 (0.5071, 12.1768) -> (0.5071, 12.4949)
  line L483 (0.5071, 12.4949) -> (-1.4823, 12.4949)
  line L484 (-1.4823, 12.4949) -> (-1.4823, 12.1768)
  line L485 (-1.4823, 12.1768) -> (-1.7376, 12.1768)
  line L486 (-1.7376, 12.1768) -> (-1.7376, 13.1452)
  line L487 (-1.7376, 13.1452) -> (-1.4823, 13.1452)
  line L488 (-1.4823, 13.1452) -> (-1.4823, 12.8271)
  line L489 (-1.4823, 12.8271) -> (0.5071, 12.8271)
  line L490 (0.5071, 12.8271) -> (0.5071, 13.1452)
  line L491 (0.5071, 13.1452) -> (0.7624, 13.1452)
  line L492 (0.7624, 15.3454) -> (0.7624, 14.9726)
  line L493 (0.7624, 14.9726) -> (-1.3932, 13.8664)
  line L494 (-1.3932, 13.8664) -> (0.7624, 13.8664)
  line L495 (0.7624, 13.8664) -> (0.7624, 13.5565)
  line L496 (0.7624, 13.5565) -> (-1.7376, 13.5565)
  line L497 (-1.7376, 13.5565) -> (-1.7376, 14.0285)
  line L498 (-1.7376, 14.0285) -> (0.2417, 15.0354)
  line L499 (0.2417, 15.0354) -> (-1.7376, 15.0354)
  line L500 (-1.7376, 15.0354) -> (-1.7376, 15.3454)
  line L501 (-1.7376, 15.3454) -> (0.7624, 15.3454)
  line L502 (3.4624, 12.4989) -> (3.4624, 12.1667)
  line L503 (3.4624, 12.1667) -> (1.3088, 12.1667)
  line L504 (1.3088, 12.1667) -> (2.7736, 11.5143)
  line L505 (2.7736, 11.5143) -> (2.7736, 11.3117)
  line L506 (2.7736, 11.3117) -> (1.3088, 10.6655)
  line L507 (1.3088, 10.6655) -> (3.4624, 10.6655)
  line L508 (3.4624, 10.6655) -> (3.4624, 10.3555)
  line L509 (3.4624, 10.3555) -> (0.9624, 10.3555)
  line L510 (0.9624, 10.3555) -> (0.9624, 10.8093)
  line L511 (0.9624, 10.8093) -> (2.3542, 11.4333)
  line L512 (2.3542, 11.4333) -> (0.9624, 12.037)
  line L513 (0.9624, 12.037) -> (0.9624, 12.4989)
  line L514 (0.9624, 12.4989) -> (3.4624, 12.4989)
  spline S453 degree 2 poles (1.2481, 14.774) (1.4142, 14.9159) (1.9004, 15.0739) (2.2124, 15.0739) knots 0 0 0 1 2 2 2
  spline S454 degree 2 poles (2.2124, 15.0739) (2.5163, 15.0739) (3.0086, 14.9199) (3.1747, 14.774) knots 0 0 0 1 2 2 2
  spline S455 degree 2 poles (3.1747, 14.774) (3.349, 14.6201) (3.5151, 14.2129) (3.5151, 13.9677) knots 0 0 0 1 2 2 2
  spline S456 degree 2 poles (3.5151, 13.9677) (3.5151, 13.7145) (3.3429, 13.3093) (3.1747, 13.1614) knots 0 0 0 1 2 2 2
  spline S457 degree 2 poles (3.1747, 13.1614) (3.0086, 13.0176) (2.5204, 12.8636) (2.2124, 12.8636) knots 0 0 0 1 2 2 2
  spline S458 degree 2 poles (2.2124, 12.8636) (1.8984, 12.8636) (1.4203, 13.0196) (1.2481, 13.1634) knots 0 0 0 1 2 2 2
  spline S459 degree 2 poles (1.2481, 13.1634) (1.0819, 13.3093) (0.9097, 13.7165) (0.9097, 13.9677) knots 0 0 0 1 2 2 2
  spline S460 degree 2 poles (0.9097, 13.9677) (0.9097, 14.223) (1.088, 14.6322) (1.2481, 14.774) knots 0 0 0 1 2 2 2
  spline S461 degree 2 poles (2.2124, 14.7274) (1.9652, 14.7274) (1.5823, 14.6201) (1.4567, 14.5228) knots 0 0 0 1 2 2 2
  spline S462 degree 2 poles (1.4567, 14.5228) (1.3271, 14.4236) (1.1974, 14.144) (1.1974, 13.9698) knots 0 0 0 1 2 2 2
  spline S463 degree 2 poles (1.1974, 13.9698) (1.1974, 13.7894) (1.323, 13.518) (1.4567, 13.4146) knots 0 0 0 1 2 2 2
  spline S464 degree 2 poles (1.4567, 13.4146) (1.5844, 13.3154) (1.9693, 13.21) (2.2124, 13.21) knots 0 0 0 1 2 2 2
  spline S465 degree 2 poles (2.2124, 13.21) (2.7047, 13.21) (3.2274, 13.6233) (3.2274, 13.9698) knots 0 0 0 1 2 2 2
  spline S466 degree 2 poles (3.2274, 13.9698) (3.2274, 14.3162) (2.7047, 14.7274) (2.2124, 14.7274) knots 0 0 0 1 2 2 2
  spline S467 degree 2 poles (2.2144, 17.4098) (2.5568, 17.4098) (3.1079, 17.1322) (3.2618, 16.8992) knots 0 0 0 1 2 2 2
  spline S468 degree 2 poles (3.2618, 16.8992) (3.3814, 16.7088) (3.4624, 16.3178) (3.4624, 16.0139) knots 0 0 0 1 2 2 2
  line L515 (3.4624, 16.0139) -> (3.4624, 15.4386)
  line L516 (3.4624, 15.4386) -> (0.9624, 15.4386)
  line L517 (0.9624, 15.4386) -> (0.9624, 16.0078)
  spline S469 degree 2 poles (0.9624, 16.0078) (0.9624, 16.3604) (1.0678, 16.7615) (1.161, 16.9033) knots 0 0 0 1 2 2 2
  spline S470 degree 2 poles (1.161, 16.9033) (1.321, 17.1444) (1.8498, 17.4098) (2.2144, 17.4098) knots 0 0 0 1 2 2 2
  spline S471 degree 2 poles (2.2104, 17.0633) (1.9227, 17.0633) (1.5155, 16.8729) (1.4, 16.6845) knots 0 0 0 1 2 2 2
  spline S472 degree 2 poles (1.4, 16.6845) (1.321, 16.5508) (1.2501, 16.2489) (1.2501, 16.024) knots 0 0 0 1 2 2 2
  line L518 (1.2501, 16.024) -> (1.2501, 15.7708)
  line L519 (1.2501, 15.7708) -> (3.1747, 15.7708)
  line L520 (3.1747, 15.7708) -> (3.1747, 16.024)
  spline S473 degree 2 poles (3.1747, 16.024) (3.1747, 16.2449) (3.1038, 16.5792) (3.0086, 16.7149) knots 0 0 0 1 2 2 2
  spline S474 degree 2 poles (3.0086, 16.7149) (2.8911, 16.8891) (2.5021, 17.0633) (2.2104, 17.0633) knots 0 0 0 1 2 2 2
  point P0 (0, 0)
  constraints: 12 other
extrude "Extrusion2" add sketch "Sketch2" along normal blind 0.5
fillet "Fillet2" radius 1 4 edges at (-13.0046, 19.6218, 0.4) (-13.0046, -19.6218, 0.4) (13.0139, -19.6218, 0.4) (13.0139, 19.6218, 0.4)
body "Solid1"
